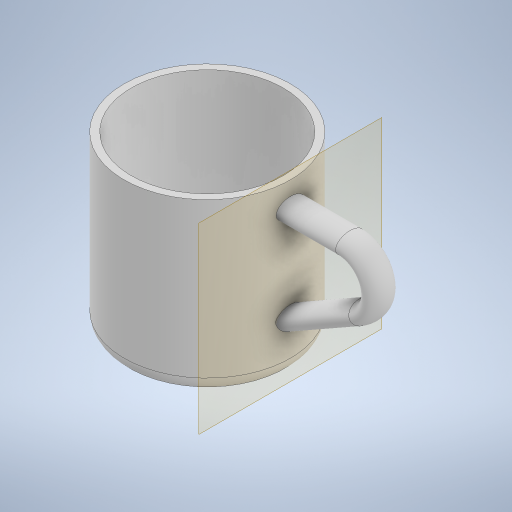
# Autodesk Inventor part: Taza de Dinamica
Saved by Autodesk Inventor 2024 (Build 280153000, 153)
## iProperties
Created: 2024-02-18
Part Number: Taza de Dinamica
Material: Genérico
Document SubType Name: Modeling
Designer: Eva Sinay
Density: 1 g/cm^3
Appearance: Valor por defecto
Author: Eva Sinay
Autodesk Inventor part; units mm, degrees
ref_plane "XZ Plane" through (0, 0, 0) normal (0, 1, 0) x (-1, 0, 0)
ref_plane "XY Plane" through (0, 0, 0) normal (0, 0, 1) x (1, 0, 0)
sketch "Boceto1" plane through (0, 0, 0) normal (0, 0, 1) x (1, 0, 0)
  line L0 (0, 0) -> (0, 70)
  line L1 (0, 70) -> (-35, 70)
  line L2 (-35, 70) -> (-35, 5)
  line L3 (0, 0) -> (-32.5, 0)
  arc A0 (-35, 5) -> (-32.5, 0) centre (-28.75, 5) ccw
  constraints: 8 end point, 2 horizontal, 2 point on circle, 1 centre point, 1 perpendicular, 1 vertical
revolve "Revolución1" add sketch "Boceto1" angle 360 about axis through (0, 0, 0) along (0, 1, 0)
shell "Vaciado1" thickness 3 removed faces 1 at (-0.2748, 70, -9.3581)
sketch "Boceto2" plane through (0, 0, 0) normal (0, 0, 1) x (1, 0, 0)
  line L0 (35, 70) -> (-35, 70) projected
  line L1 (35, 5) -> (35, 70) projected
  line L2 (35, 60) -> (60, 60)
  line L3 (35, 5) -> (-35, 5) projected
  line L4 (35, 20) -> (65.8095, 37.5)
  arc A0 (65.8095, 37.5) -> (60, 60) centre (60, 48) ccw
  point P0 (0, 0)
  dimension "d11" = 10
  dimension "d13" = 15
  dimension "d16" = 12
  constraints: 4 end point, 2 point on circle, 2 point on line, 1 centre point
  measures "d11" distance of L1.end L2.start
  measures "d13" distance of L1.start L4.start
  measures "d16" radius of A0
ref_plane "Plano de trabajo1" through (35, 60, 0) normal (1, 0, 0) x (0, 1, 0)
sketch "Boceto4" plane through (35, 60, 0) normal (1, 0, 0) x (0, 1, 0)
  ellipse E0 centre (-39.9635, 0) end of major axis (-39.9635, 5) minor radius 3
  ellipse E1 centre (0, 0) end of major axis (0, -6) minor radius 4
  point P0 (-60, 0)
  dimension "d17" = 3
  dimension "d18" = 5
  dimension "d19" = 4
  dimension "d20" = 6
  constraints: 4 other
sweep "Barrido1" add profiles "Boceto4" path "Boceto2" path curves L2 A0 L4 contours E1
